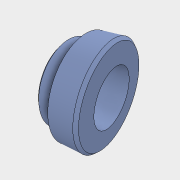
# Autodesk Inventor part: Collar
Saved by Autodesk Inventor 2020.1 (Build 241239000, 239)
## iProperties
Created: 2019-09-11
Part Number: Collar
Material: Nylon 6/6
Document SubType Name: Modeling
Designer: thom_tremblay
Density: 1.13 g/cm^3
Appearance: Rubber - Blue
Author: thom_tremblay
Autodesk Inventor part; units mm, degrees
ref_plane "YZ Plane" through (0, 0, 0) normal (1, 0, 0) x (0, 1, 0)
ref_plane "XZ Plane" through (0, 0, 0) normal (0, 1, 0) x (-1, 0, 0)
ref_plane "XY Plane" through (0, 0, 0) normal (0, 0, 1) x (1, 0, 0)
sketch "Sketch1" plane through (0, 0, 0) normal (0, 1, 0) x (-1, 0, 0)
  line L0 (0, 0) -> (0, -25.0217)
  line L1 (-12.827, 0) -> (-18.923, 0)
  line L2 (-18.923, 0) -> (-18.923, -20.32)
  line L3 (-18.923, -20.32) -> (-12.827, -20.32)
  line L4 (-12.827, -20.32) -> (-12.827, 0)
  line L5 (-18.923, -20.32) -> (-22.86, -20.32)
  line L6 (-22.86, -20.32) -> (-22.86, -8.89)
  line L7 (-22.86, -8.89) -> (-18.923, -8.89)
  line L8 (-18.923, -8.89) -> (-18.923, -20.32)
  dimension "d0" = 25.654
  dimension "d1" = 20.32
  dimension "d2" = 8.89
  dimension "d3" = 37.846
  dimension "d4" = 45.72
  constraints: 18 end point, 4 parallel, 2 horizontal, 2 perpendicular, 1 horizontal alignment, 1 vertical
  measures "d0" diameter of L4 L0
  measures "d1" distance of L1.end L2.end
  measures "d2" distance between parallel lines of L7 L1
  measures "d3" diameter of L2 L0
  measures "d4" diameter of L6 L0
revolve "Revolution1" add sketch "Sketch1" angle 360 about axis through (0, 0, 0) along (0, 0, -1)
chamfer "Chamfer1" distance 1.27 angle 45 2 edges at (-18.923, 0, 0) (-22.86, 0, -20.32)
body "Solid1"
